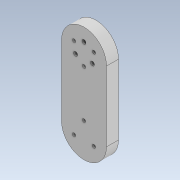
# Autodesk Inventor part: shank_thigh_connector
Saved by Autodesk Inventor 2020 (Build 240168000, 168)
## iProperties
Created: 2021-01-06
Part Number: shank_thigh_connector
Material: Generic
Document SubType Name: Modeling
Designer: DELL
Density: 1 g/cm^3
Appearance: Default
Author: DELL
Autodesk Inventor part; units mm, degrees
ref_plane "YZ Plane" through (0, 0, 0) normal (1, 0, 0) x (0, 1, 0)
ref_plane "XZ Plane" through (0, 0, 0) normal (0, 1, 0) x (-1, 0, 0)
ref_plane "XY Plane" through (0, 0, 0) normal (0, 0, 1) x (1, 0, 0)
sketch "Sketch1" plane through (0, 0, 0) normal (0, 0, 1) x (1, 0, 0)
  circle A0 centre (0, 0) radius 22.5
  circle A1 centre (0, -70) radius 22.5
  line L0 (-22.5, 0) -> (-22.5, -70)
  line L1 (22.5, 0) -> (22.5, -70)
  circle A2 centre (0, -70) radius 11.5 construction
  circle A3 centre (0, -70) radius 9.715 construction
  line L2 (0, -20) -> (0, -150) construction
  line L3 (11.5, -70) -> (-11.5, -70) construction
  line L4 (9.9593, -64.25) -> (0, -70) construction
  line L5 (0, -70) -> (-9.9593, -64.25) construction
  line L6 (0, -70) -> (9.9593, -75.75) construction
  line L7 (0, -70) -> (-9.9593, -75.75) construction
  circle A4 centre (0, -58.5) radius 2.75
  circle A5 centre (9.9593, -75.75) radius 2.75
  circle A6 centre (-9.9593, -75.75) radius 2.75
  circle A7 centre (0, -58.5) radius 1.65
  circle A8 centre (9.9593, -75.75) radius 1.65
  circle A9 centre (-9.9593, -75.75) radius 1.65
  circle A10 centre (8.4134, -65.1425) radius 2
  circle A11 centre (0, -79.715) radius 2
  circle A12 centre (-8.4134, -65.1425) radius 2
  line L8 (-22.5, -35) -> (22.5, -35) construction
  circle A13 centre (0, 0) radius 22.5
  line L9 (9.9593, -5.75) -> (0, 0) construction
  circle A14 centre (8.4134, -4.8575) radius 2
  line L10 (0, 0) -> (9.9593, 5.75) construction
  line L11 (0, 0) -> (-9.9593, -5.75) construction
  circle A15 centre (-8.4134, -4.8575) radius 2
  circle A16 centre (0, 0) radius 9.715 construction
  circle A17 centre (0, 0) radius 11.5 construction
  circle A18 centre (0, 9.715) radius 2
  line L12 (0, 0) -> (-9.9593, 5.75) construction
  line L13 (11.5, 0) -> (-11.5, 0) construction
  circle A19 centre (-9.9593, 5.75) radius 2.75
  circle A20 centre (-9.9593, 5.75) radius 1.65
  line L14 (0, -50) -> (0, 80) construction
  circle A21 centre (0, -11.5) radius 1.65
  circle A22 centre (0, -11.5) radius 2.75
  circle A23 centre (9.9593, 5.75) radius 2.75
  circle A24 centre (9.9593, 5.75) radius 1.65
  dimension "d3" = 23
  dimension "d0" = 45
  dimension "d1" = 70
  dimension "d2" = 19.43
  dimension "d4" = 30
  dimension "d5" = 30
  dimension "d6" = 30
  dimension "d7" = 30
  dimension "d8" = 5.5
  dimension "d9" = 3.3
  dimension "d10" = 4
  constraints: 30 end point, 23 centre point, 22 symmetric about line, 17 coincident, 10 point on circle, 10 point on line, 7 equal radius, 5 midpoint, 4 tangent, 2 horizontal, 2 vertical alignment, 29 other
  measures "d0" diameter of A0
  measures "d1" distance of L1.start L1.end
  measures "d2" diameter of A3
  measures "d4" angle of L3 L4
  measures "d5" angle of L3 L6
  measures "d6" angle of L3 L5
  measures "d7" angle of L3 L7
  measures "d8" diameter of A4
  measures "d9" diameter of A7
  measures "d10" diameter of A10
extrude "Extrusion1" add sketch "Sketch1" along normal blind 12 contours A0 | L1 A1 L0 A0 | A1 | A4 | A5 | A6 | A10 | A11 | A12 | A14 | A15 | A18 | A19 | A22 | A23
extrude "Extrusion2" cut sketch "Sketch1" along normal blind 5 contours A4 | A5 | A6 | A19 | A22 | A23 | A24
extrude "Extrusion3" cut sketch "Sketch1" against normal blind 5 from surface at 12 contours A14 | A15 | A18
body "Solid1"
